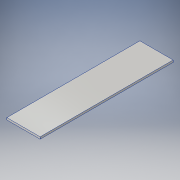
# Autodesk Inventor part: longSupportPlate
Saved by Autodesk Inventor 2016 SP1 (Build 200210100, 210)
## iProperties
Created: 2016-02-05
Part Number: longSupportPlate
Material: Aluminum 6061
Document SubType Name: Modeling
Designer: steele
Density: 2.7 g/cm^3
Appearance: Aluminum - Flat
Mass: 707.921 g
Surface Area: 890.321 cm^2
Volume: 262.193 cm^3
Author: steele
Autodesk Inventor part; units mm, degrees
ref_plane "YZ Plane" through (0, 0, 0) normal (1, 0, 0) x (0, 1, 0)
ref_plane "XZ Plane" through (0, 0, 0) normal (0, 1, 0) x (-1, 0, 0)
ref_plane "XY Plane" through (0, 0, 0) normal (0, 0, 1) x (1, 0, 0)
sketch "Sketch1" plane through (0, 0, 0) normal (0, 1, 0) x (-1, 0, 0)
  line L0 (50.8, 203.2) -> (-50.8, 203.2)
  line L1 (-50.8, 203.2) -> (-50.8, -203.2)
  line L2 (-50.8, -203.2) -> (50.8, -203.2)
  line L3 (50.8, -203.2) -> (50.8, 203.2)
  line L4 (50.8, 203.2) -> (-50.8, -203.2) construction
  line L5 (-50.8, 203.2) -> (50.8, -203.2) construction
  point P0 (0, 0)
  dimension "d0" = 406.4
  dimension "d1" = 101.6
  constraints: 12 end point, 2 midpoint, 2 parallel, 1 horizontal, 1 perpendicular
  measures "d0" distance of L2.end L0.start
  measures "d1" distance of L0.start L0.end
extrude "Extrusion1" add sketch "Sketch1" along normal blind 6.35
equation "\"d0\" = plateLength"
equation "\"d1\" = plateWidth"
equation "\"d2\" = plateThickness"
equation "\"plateWidth\" = 101.6"
equation "\"plateLength\" = 406.4"
equation "\"plateThickness\" = 6.35"
body "Solid1"
